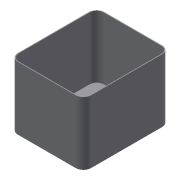
# Autodesk Inventor part: speaker body
Saved by Autodesk Inventor 2014 (Build 180170000, 170)
## iProperties
Created: 2015-10-11
Part Number: speaker body
Material: Generic
Document SubType Name: Modeling
Designer: Devon
Density: 1 g/cm^3
Appearance: Default
Author: Devon
Autodesk Inventor part; units mm, degrees
ref_plane "YZ Plane" through (0, 0, 0) normal (1, 0, 0) x (0, 1, 0)
ref_plane "XZ Plane" through (0, 0, 0) normal (0, 1, 0) x (-1, 0, 0)
ref_plane "XY Plane" through (0, 0, 0) normal (0, 0, 1) x (1, 0, 0)
sketch "Sketch1" plane through (0, 0, 0) normal (0, 1, 0) x (-1, 0, 0)
  line L0 (-4.439, 1.111) -> (42.678, 1.111)
  line L1 (49.028, -5.239) -> (49.028, -63.151)
  line L2 (42.678, -69.501) -> (-4.439, -69.501)
  line L3 (-10.789, -63.151) -> (-10.789, -5.239)
  arc A0 (49.028, -5.239) -> (42.678, 1.111) centre (42.678, -5.239) ccw
  arc A1 (42.678, -69.501) -> (49.028, -63.151) centre (42.678, -63.151) ccw
  arc A2 (-10.789, -63.151) -> (-4.439, -69.501) centre (-4.439, -63.151) ccw
  arc A3 (-4.439, 1.111) -> (-10.789, -5.239) centre (-4.439, -5.239) ccw
  point P0 (0, 0)
  point P1 (49.028, -69.501)
  point P2 (49.028, 1.111)
  point P3 (-10.789, -69.501)
  dimension "d0" = 59.817
  dimension "d1" = 70.612
  dimension "d2" = 6.35
  constraints: 8 end point, 8 point on circle, 8 tangent, 6 point on line, 4 centre point, 3 equal radius, 2 parallel, 1 horizontal, 1 perpendicular
  measures "d0" distance of point (49.028, -69.501) point (-10.789, -69.501)
  measures "d1" distance of point (49.028, 1.111) point (49.028, -69.501)
  measures "d2" radius of A0
extrude "Extrusion1" add sketch "Sketch1" along normal blind 0.635
sketch "Sketch2" plane through (0, 0.635, 0) normal (0, 1, 0) x (1, 0, 0)
  line L0 (-49.028, 63.151) -> (-49.028, 5.239) projected
  arc A0 (-49.028, 5.239) -> (-42.678, -1.111) centre (-42.678, 5.239) ccw projected
  line L1 (-42.678, -1.111) -> (4.439, -1.111) projected
  arc A1 (4.439, -1.111) -> (10.789, 5.239) centre (4.439, 5.239) ccw projected
  line L2 (10.789, 5.239) -> (10.789, 63.151) projected
  arc A2 (10.789, 63.151) -> (4.439, 69.501) centre (4.439, 63.151) ccw projected
  line L3 (4.439, 69.501) -> (-42.678, 69.501) projected
  arc A3 (-42.678, 69.501) -> (-49.028, 63.151) centre (-42.678, 63.151) ccw projected
  line L4 (-19.1195, 68.866) -> (4.439, 68.866)
  line L5 (10.154, 34.195) -> (10.154, 63.151)
  line L6 (-19.1195, -0.476) -> (4.439, -0.476)
  line L7 (-48.393, 34.195) -> (-48.393, 63.151)
  line L8 (-19.1195, 68.866) -> (-42.678, 68.866)
  line L9 (-48.393, 34.195) -> (-48.393, 5.239)
  line L10 (-19.1195, -0.476) -> (-42.678, -0.476)
  line L11 (10.154, 34.195) -> (10.154, 5.239)
  arc A4 (-42.678, 68.866) -> (-48.393, 63.151) centre (-42.678, 63.151) ccw
  arc A5 (10.154, 63.151) -> (4.439, 68.866) centre (4.439, 63.151) ccw
  arc A6 (4.439, -0.476) -> (10.154, 5.239) centre (4.439, 5.239) ccw
  arc A7 (-48.393, 5.239) -> (-42.678, -0.476) centre (-42.678, 5.239) ccw
  point P0 (0, 0)
  dimension "d9" = 5.715
  dimension "d10" = 5.715
  constraints: 16 end point, 8 point on circle, 8 tangent, 5 perpendicular, 4 centre point, 2 equal radius
  measures "d9" radius of A4
  measures "d10" radius of A5
extrude "Extrusion2" add sketch "Sketch2" along normal blind 50.8
body "Solid1"
